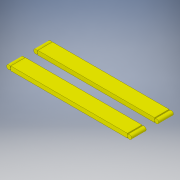
# Autodesk Inventor part: elev1
Saved by Autodesk Inventor 2016 (Build 200138000, 138)
## iProperties
Created: 2018-01-10
Part Number: elev1
Material: Aluminum 6061
Document SubType Name: Modeling
Designer: New User
Density: 2.7 g/cm^3
Appearance: Aluminum - Flat
Mass: 9160.72 g
Surface Area: 3667.5 cm^2
Volume: 3392.86 cm^3
Author: New User
Autodesk Inventor part; units mm, degrees
ref_plane "YZ Plane" through (0, 0, 0) normal (1, 0, 0) x (0, 1, 0)
ref_plane "XZ Plane" through (0, 0, 0) normal (0, 1, 0) x (-1, 0, 0)
ref_plane "XY Plane" through (0, 0, 0) normal (0, 0, 1) x (1, 0, 0)
sketch "Sketch1" plane through (0, 0, 0) normal (0, 1, 0) x (-1, 0, 0)
  line L0 (0, 0) -> (711.2, 0)
  line L1 (711.2, 0) -> (711.2, 88.9)
  line L2 (711.2, 88.9) -> (0, 88.9)
  line L3 (0, 88.9) -> (0, 0)
  line L4 (711.2, -76.2) -> (0, -76.2)
  line L5 (0, -76.2) -> (0, -165.1)
  line L6 (0, -165.1) -> (711.2, -165.1)
  line L7 (711.2, -165.1) -> (711.2, -76.2)
  dimension "d0" = 88.9
  dimension "d1" = 711.2
  dimension "d2" = 88.9
  dimension "d3" = 711.2
  dimension "d4" = 76.2
  constraints: 16 end point, 4 parallel, 2 horizontal, 2 perpendicular
  measures "d0" distance of L2.end L0.start
  measures "d1" distance of L1.end L2.end
  measures "d2" distance of L4.end L5.end
  measures "d3" distance of L5.end L6.end
  measures "d4" distance between parallel lines of L4 L0
extrude "Extrusion1" add sketch "Sketch1" along normal blind 25.4
sketch "Sketch2" plane through (-711.2, 0, -76.2) normal (0, 0, 1) x (1, 0, 0)
  line L0 (0, 25.4) -> (711.2, 25.4) projected
  circle A0 centre (723.9, 12.7) radius 12.7
  line L1 (711.2, 0) -> (0, 0) projected
  circle A1 centre (-12.7, 12.7) radius 12.7
  constraints: 2 centre point
extrude "Extrusion4" add sketch "Sketch2" along normal blind 165.1 and the other way blind 89.7001
sketch "Sketch3" plane through (0, 25.4, 88.9) normal (1, 0, 0) x (0, 0, -1)
  line L0 (88.9, -37.8138) -> (165.1, -37.8138)
  line L1 (165.1, -37.8138) -> (165.1, 10.1358)
  line L2 (165.1, 10.1358) -> (88.9, 10.1358)
  line L3 (88.9, 10.1358) -> (88.9, -37.8138)
  point P0 (88.9, -25.4)
  constraints: 8 end point, 2 parallel, 1 horizontal, 1 perpendicular
extrude "Extrusion3" cut sketch "Sketch3" along normal blind 68.2625 and the other way blind 827.8876
body "Solid1"
